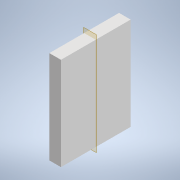
# Autodesk Inventor part: sideSupportFor-12inch
Saved by Autodesk Inventor 2021 (Build 250183000, 183)
## iProperties
Created: 2020-07-01
Part Number: sideSupportFor-12inch
Material: Generic
Document SubType Name: Modeling
Designer: robst
Density: 1 g/cm^3
Appearance: Default
Author: robst
Autodesk Inventor part; units mm, degrees
ref_plane "YZ Plane" through (0, 0, 0) normal (1, 0, 0) x (0, 1, 0)
ref_plane "XZ Plane" through (0, 0, 0) normal (0, 1, 0) x (-1, 0, 0)
ref_plane "XY Plane" through (0, 0, 0) normal (0, 0, 1) x (1, 0, 0)
sketch "Sketch1" plane through (0, 0, 0) normal (0, 1, 0) x (-1, 0, 0)
  line L0 (12.7, 76.2) -> (-12.7, 76.2)
  line L1 (-12.7, 76.2) -> (-12.7, -76.2)
  line L2 (-12.7, -76.2) -> (12.7, -76.2)
  line L3 (12.7, -76.2) -> (12.7, 76.2)
  line L4 (12.7, 76.2) -> (-12.7, -76.2) construction
  line L5 (-12.7, 76.2) -> (12.7, -76.2) construction
  point P0 (0, 0)
  dimension "d0" = 25.4
  dimension "d1" = 152.4
  constraints: 12 end point, 2 midpoint, 2 parallel, 1 horizontal, 1 perpendicular
  measures "d0" distance of L0.start L0.end
  measures "d1" distance of L2.end L0.start
extrude "Extrusion1" add sketch "Sketch1" along normal blind 203.2
sketch "Sketch2" plane through (-12.7, 0, -76.2) normal (-1, 0, 0) x (0, 0, 1)
  line L0 (152.4, 203.2) -> (0, 203.2) construction
  line L1 (76.2, 203.2) -> (76.2, 0) construction
  circle A0 centre (76.2, 177.8) radius 12.7
  dimension "d4" = 25.4
  dimension "d7" = 25.4
  constraints: 2 end point, 1 centre point, 1 midpoint, 1 point on line, 1 vertical
  measures "d4" diameter of A0
  measures "d7" distance from line of A0.centre L0
extrude "Extrusion2" cut sketch "Sketch2" against normal through all
body "Solid1"
